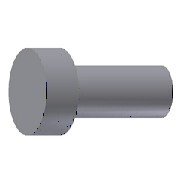
# Autodesk Inventor part: AH 1.5 -200
Saved by Autodesk Inventor 2024 (Build 280153000, 153)
## iProperties
IsCustomPart: 1
Created: 2023-01-19
Part Number: AH 1.5 -200
Material: DIN 1.2210
Description: Ejector pins-hardened
Document SubType Name: Modeling
Standard: DIN 1530/ISO 6751
Designer: Alex
Standard Revision: 1
Manufacturer: DME
Language: en-US
Size Designation: 1.5 -200
Categories: <MemberInstance><Categories><Category DisplayName="Mold" InternalName="349578f2-f4d4-4954-8c09-8e99297a61c0" Mnemonic="MOLD"><Category DisplayName="Ejector Components" InternalName="a65bc7a0-4d93-4421-bfd9-68036df3df42" Mnemonic="EJECTOR COMPONENTS"><Category DisplayName="Ejector Pins" InternalName="7afbd714-7cef-4652-97a0-e763dbf62ebd" Mnemonic="EJECTOR PINS"><CategoryParameter DisplayName="Nominal Length" InternalName="5cc51ba1-9638-47ad-aa8b-04b28756f61b" Mnemonic="NOMINAL LENGTH"/><CategoryParameter DisplayName="Head Diameter" InternalName="c3327d1f-5c0c-452b-9f22-1276b220c59f" Mnemonic="HEAD DIAMETER"/><CategoryParameter DisplayName="Head Height" InternalName="c72c4b8c-fb82-4099-a813-f68e4c711a7f" Mnemonic="HEAD HEIGHT"/><Category DisplayName="Straight" InternalName="5bbfdb80-b444-4b08-9ee6-a4b602cc2e17" Mnemonic="STRAIGHT"><CategoryParameter DisplayName="Anti-rotary Plane Width" InternalName="0465766b-1a49-41ec-91b0-1525f149beb7" Mnemonic="ANTI-ROTARY PLANE WIDTH"/><CategoryParameter DisplayName="Nominal Diameter" InternalName="75e7570f-bb9b-4b2d-a4cd-5226cced53dc" Mnemonic="NOMINAL DIAMETER"/><CategoryParameter DisplayName="Anti-rotary Hole Diameter" InternalName="eee4f5a1-5f5f-432c-942f-281c4b20c6a1" Mnemonic="ANTI-ROTARY HOLE DIAMETER"/></Category></Category></Category></Category><Category DisplayName="DataType" InternalName="23b78d0f-2648-40c6-8793-ca6db495c9e8" Mnemonic="DATATYPE"><CategoryParameter DisplayName="DisplayName" InternalName="05415f3d-3907-474b-a020-eb9d644f4cf3" Mnemonic="DISPLAYNAME"/><CategoryParameter DisplayName="Standard" InternalName="0c0a119c-1e12-4c84-803f-101930972f5e" Mnemonic="STANDARD"/><CategoryParameter DisplayName="Description" InternalName="13903e3d-64b1-4950-80da-f627842ea37f" Mnemonic="DESCRIPTION"/><CategoryParameter DisplayName="Designation" InternalName="2675968c-4ce5-49e0-a4f5-552d29089031" Mnemonic="DESIGNATION"/><CategoryParameter DisplayName="Default Row" InternalName="2af9ec52-faaa-4026-b378-f9fa4afca842" Mnemonic="DEFAULTROW"/><CategoryParameter DisplayName="Folder Name" InternalName="3f06958e-8713-4116-9be7-ed6184ecc97b" Mnemonic="FOLDERNAME"/><CategoryParameter DisplayName="Revision Guid" InternalName="45a75005-10b1-4dfc-8d6d-dfe629f0b93c" Mnemonic="REVISIONGUID"/><CategoryParameter DisplayName="FileName" InternalName="8b46a4cc-9585-4fed-90c3-899f57e09a73" Mnemonic="FILENAME"/><CategoryParameter DisplayName="StdsOrg" InternalName="8f5914e1-4693-403f-8ab5-d37768198c9d" Mnemonic="STDSORG"/><CategoryParameter DisplayName="Family Version" InternalName="914462f6-6e19-4b14-ba84-155b9680b1d0" Mnemonic="FAMILYREVISION"/><CategoryParameter DisplayName="Standard Revision" InternalName="91d5a463-65c2-4fde-b823-3b7fea5e8e17" Mnemonic="STANDARDREVISION"/><CategoryParameter DisplayName="Member Revision" InternalName="a65d44b9-392f-4f4f-857b-e4b3d54996fe" Mnemonic="MEMBERREVISION"/><CategoryParameter DisplayName="ClipFormat" InternalName="bc51e27b-3422-4e78-93ef-cec197ddf230" Mnemonic="CLIPFORMAT"/><CategoryParameter DisplayName="Manufacturer" InternalName="cd6c7a72-a28a-4e50-99a9-2c7f4e13e5ad" Mnemonic="MANUFACTURER"/><CategoryParameter DisplayName="InternalName" InternalName="cf1d0246-76d9-4b4a-8305-fa0409afb5c1" Mnemonic="INTERNALNAME"/><CategoryParameter DisplayName="IsMetric" InternalName="e2385c5b-1ea4-4823-96a8-8de651266ec3" Mnemonic="ISMETRIC"/><Category DisplayName="Part" InternalName="c0e0b642-3bcb-4cc8-9e80-f96d35c4afa4" Mnemonic="PART"><CategoryParameter DisplayName="Part Number" InternalName="016b6077-bfbe-49bd-92c9-d8d59c39c941" Mnemonic="PARTNUMBER"/><CategoryParameter DisplayName="Stock Number" InternalName="4dba7c1c-e26c-444e-836c-b08b433409a8" Mnemonic="STOCKNUMBER"/><CategoryParameter DisplayName="Material Key" InternalName="5c9a8adb-dd2b-4535-b97f-0a94a95fe41f" Mnemonic="MATERIALKEY"/><CategoryParameter DisplayName="Material" InternalName="818a152a-d3c3-49ca-80ee-df7d91421b8e" Mnemonic="MATERIAL"/></Category></Category></Categories><FamilyTemplate Id="AH"><FamilyTemplateParameters><FamilyTemplateParameter ObjectType="kUserParameterObject" ValueType="xs:double" Id="1" ObjectReferenceKey="L"/><FamilyTemplateParameter ObjectType="kUserParameterObject" ValueType="xs:double" Id="2" ObjectReferenceKey="R"/><FamilyTemplateParameter ObjectType="kUserParameterObject" ValueType="xs:double" Id="3" ObjectReferenceKey="T_"/><FamilyTemplateParameter ObjectType="kUserParameterObject" ValueType="xs:double" Id="4" ObjectReferenceKey="H_"/><FamilyTemplateParameter ObjectType="kUserParameterObject" ValueType="xs:double" Id="5" ObjectReferenceKey="P"/><FamilyTemplateParameter ObjectType="kUserParameterObject" ValueType="xs:double" Id="6" ObjectReferenceKey="Anti_Rotary_D"/><FamilyTemplateParameter ObjectType="kUserParameterObject" ValueType="xs:double" Id="7" ObjectReferenceKey="Anti_Rotary_P"/><FamilyTemplateParameter ObjectType="kPartComponentDefinitionObject" ValueType="xs:string" Id="8" SubObjectId="Material"/><FamilyTemplateParameter ObjectType="kPropertyObject" ValueType="xs:string" Id="17" ObjectReferenceKey="{32853F0F-3444-11d1-9E93-0060B03C1CA6}" SubObjectId="5"/><FamilyTemplateParameter ObjectType="kPropertyObject" ValueType="xs:string" Id="18" ObjectReferenceKey="{32853F0F-3444-11d1-9E93-0060B03C1CA6}" SubObjectId="52"/></FamilyTemplateParameters></FamilyTemplate><CategoryParameterMap><ParamToTemplateMap><ParamToTemplate CategoryParameter="//CategoryParameter[@InternalName='2af9ec52-faaa-4026-b378-f9fa4afca842']" ConstantValue="1"/><ParamToTemplate CategoryParameter="//CategoryParameter[@InternalName='bc51e27b-3422-4e78-93ef-cec197ddf230']" ConstantValue="CF_INVENTOR.STDPARTS"/><ParamToTemplate CategoryParameter="//CategoryParameter[@InternalName='e2385c5b-1ea4-4823-96a8-8de651266ec3']" ConstantValue="true"/><ParamToTemplate CategoryParameter="//CategoryParameter[@InternalName='cf1d0246-76d9-4b4a-8305-fa0409afb5c1']" ConstantValue="79acf59a-664f-4cd1-ad29-20765bd07c06"/><ParamToTemplate CategoryParameter="//CategoryParameter[@InternalName='45a75005-10b1-4dfc-8d6d-dfe629f0b93c']" ConstantValue="aea4f65d-f141-4fa1-8a50-a55497a41442"/><ParamToTemplate CategoryParameter="//CategoryParameter[@InternalName='3f06958e-8713-4116-9be7-ed6184ecc97b']" ConstantValue="AH"/><ParamToTemplate CategoryParameter="//CategoryParameter[@InternalName='8f5914e1-4693-403f-8ab5-d37768198c9d']" TemplateParameter="12"/><ParamToTemplate CategoryParameter="//CategoryParameter[@InternalName='0c0a119c-1e12-4c84-803f-101930972f5e']" ConstantValue="DIN 1530/ISO 6751"/><ParamToTemplate CategoryParameter="//CategoryParameter[@InternalName='91d5a463-65c2-4fde-b823-3b7fea5e8e17']" ConstantValue="1"/><ParamToTemplate CategoryParameter="//CategoryParameter[@InternalName='cd6c7a72-a28a-4e50-99a9-2c7f4e13e5ad']" ConstantValue="DME"/><ParamToTemplate CategoryParameter="//CategoryParameter[@InternalName='13903e3d-64b1-4950-80da-f627842ea37f']" ConstantValue="Ejector pins-hardened"/><ParamToTemplate CategoryParameter="//CategoryParameter[@InternalName='05415f3d-3907-474b-a020-eb9d644f4cf3']" ConstantValue="AH"/><ParamToTemplate CategoryParameter="//CategoryParameter[@InternalName='914462f6-6e19-4b14-ba84-155b9680b1d0']" ConstantValue="1"/><ParamToTemplate CategoryParameter="//CategoryParameter[@InternalName='bc51e27b-3422-4e78-93ef-cec197ddf230']" ConstantValue="CF_INVENTOR.STDPARTS"/><ParamToTemplate CategoryParameter="//CategoryParameter[@InternalName='8b46a4cc-9585-4fed-90c3-899f57e09a73']" ConstantValue="AH 1.5 -200"/><ParamToTemplate CategoryParameter="//CategoryParameter[@InternalName='a65d44b9-392f-4f4f-857b-e4b3d54996fe']" ConstantValue="A6A251FD-8D36-48F6-BC10-C70FBE420E95"/><ParamToTemplate CategoryParameter="//CategoryParameter[@InternalName='eee4f5a1-5f5f-432c-942f-281c4b20c6a1']" TemplateParameter="6"/><ParamToTemplate CategoryParameter="//CategoryParameter[@InternalName='0465766b-1a49-41ec-91b0-1525f149beb7']" TemplateParameter="7"/><ParamToTemplate CategoryParameter="//CategoryParameter[@InternalName='2675968c-4ce5-49e0-a4f5-552d29089031']" TemplateParameter="18"/><ParamToTemplate CategoryParameter="//CategoryParameter[@InternalName='c3327d1f-5c0c-452b-9f22-1276b220c59f']" TemplateParameter="4"/><ParamToTemplate CategoryParameter="//CategoryParameter[@InternalName='5cc51ba1-9638-47ad-aa8b-04b28756f61b']" TemplateParameter="1"/><ParamToTemplate CategoryParameter="//CategoryParameter[@InternalName='818a152a-d3c3-49ca-80ee-df7d91421b8e']" TemplateParameter="8"/><ParamToTemplate CategoryParameter="//CategoryParameter[@InternalName='75e7570f-bb9b-4b2d-a4cd-5226cced53dc']" TemplateParameter="5"/><ParamToTemplate CategoryParameter="//CategoryParameter[@InternalName='016b6077-bfbe-49bd-92c9-d8d59c39c941']" TemplateParameter="17"/><ParamToTemplate CategoryParameter="//CategoryParameter[@InternalName='c72c4b8c-fb82-4099-a813-f68e4c711a7f']" TemplateParameter="3"/></ParamToTemplateMap></CategoryParameterMap></MemberInstance>
Mass: 0.191827 g
Surface Area: 2.51725 cm^2
Volume: 0.191827 cm^3
Density: 7.85 g/cm^3
Appearance: Aluminum - Dark
Author: Alex
Autodesk Inventor part; units mm, degrees
ref_plane "XZ Plane" through (0, 0, 0) normal (0, 1, 0) x (-1, 0, 0)
ref_plane "XY Plane" through (0, 0, 0) normal (0, 0, 1) x (1, 0, 0)
sketch "Sketch1" plane through (0, 0, 0) normal (0, 1, 0) x (0, 0, 1)
  line L0 (0, 1.5) -> (1.5, 1.5)
  line L1 (0, 0) -> (0, 1.5)
  line L2 (1.5, 0.75) -> (200, 0.75)
  line L3 (200, 0.75) -> (200, 0)
  line L4 (0, 0) -> (200, 0)
  line L5 (1.5, 1.5) -> (1.5, 0.75)
  point P0 (1.5, 0)
  dimension "d6" = 1.5
  dimension "d9" = 200
  dimension "d10" = 3
  dimension "d13" = 1.5
  constraints: 12 end point, 4 point on line, 2 horizontal, 2 perpendicular, 1 coincident
  measures "d6" distance of L0.start L0.end
  measures "d9" distance between parallel lines of L3 L1
  measures "d10" diameter of L0 L4
  measures "d13" diameter of L2 L4
revolve "Revolution1" add sketch "Sketch1" angle 360 about axis through (0, 0, 0) along (0, 0, 1)
fillet "Fillet1" radius 0.2 1 edges at (-0.75, 0, 1.5)
ref_plane "Work Plane1" through (1.5, 0, 0.75) normal (1, 0, 0) x (0, 1, 0)
sketch "Sketch2" plane through (1.5, 0, 0.75) normal (1, 0, 0) x (0, 1, 0)
  line L0 (1.5, -0.75) -> (-1.5, -0.75) construction
  line L1 (-1.5, -0.75) -> (-1.5, 0.75) construction
  point P0 (0, -0.75)
  point P1 (0, 0)
  point P2 (-1.5, 0)
  point P3 (0, -0.75)
  constraints: 2 midpoint, 1 horizontal alignment, 1 vertical alignment
hole "Anti_Rotary Hole" [suppressed]
sketch "Sketch3" plane through (0, 0, 0) normal (0, 0, -1) x (-1, 0, 0)
  circle A0 centre (0, 0) radius 1.5 projected
  line L0 (-1.05, 1.0712) -> (-1.05, -1.0712)
  dimension "d55" = 1.05
  constraints: 2 end point, 2 point on circle, 1 vertical
  measures "d55" distance from line of point (0, 0) L0
extrude "Anti_Rotary Plane" [suppressed]
equation "\"P\" = 1.5"
equation "\"T_\" = 1.5"
equation "\"H_\" = 3"
equation "\"R\" = 0.2"
equation "\"Anti_Rotary_P\" = 1.05"
equation "\"Anti_Rotary_D\" = 0.175"
body "Solid1"
